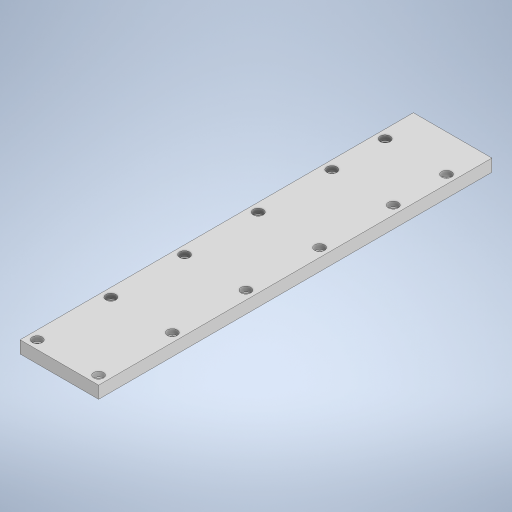
# Autodesk Inventor part: body_cover_v2
Saved by Autodesk Inventor 2023 (Build 270158000, 158)
## iProperties
Created: 2023-07-18
Part Number: body_cover_v2
Material: Generic
Document SubType Name: Modeling
Designer: checo
Density: 1 g/cm^3
Appearance: Default
Author: checo
Autodesk Inventor part; units mm, degrees
ref_plane "YZ Plane" through (0, 0, 0) normal (1, 0, 0) x (0, 1, 0)
ref_plane "XZ Plane" through (0, 0, 0) normal (0, 1, 0) x (-1, 0, 0)
ref_plane "XY Plane" through (0, 0, 0) normal (0, 0, 1) x (1, 0, 0)
sketch "Sketch1" plane through (0, 0, 0) normal (0, 1, 0) x (-1, 0, 0)
  line L0 (-16, -80.1) -> (16, -80.1)
  line L1 (16, -80.1) -> (16, 80.1)
  line L2 (16, 80.1) -> (-16, 80.1)
  line L3 (-16, 80.1) -> (-16, -80.1)
  line L4 (-16, -80.1) -> (16, 80.1) construction
  line L5 (16, -80.1) -> (-16, 80.1) construction
  point P0 (0, 0)
  dimension "d0" = 160.2
  dimension "d1" = 32
  constraints: 12 end point, 2 midpoint, 2 parallel, 1 horizontal, 1 perpendicular
  measures "d0" distance of L0.end L1.end
  measures "d1" distance of L1.end L2.end
extrude "Extrusion1" add sketch "Sketch1" along normal blind 5
sketch "Sketch2" plane through (0, 5, 0) normal (0, 1, 0) x (1, 0, 0)
  line L0 (-16, 80.1) -> (-16, -80.1) projected
  line L1 (-16, -80.1) -> (16, -80.1) projected
  line L2 (0, -80.1) -> (0, 80.1) construction
  line L3 (16, 80.1) -> (-16, 80.1) projected
  point P0 (0, 0)
  point P1 (-12.5, -76.6)
  point P2 (-12.5, -46.6)
  point P3 (-12.5, -16.6)
  point P4 (-12.5, 13.4)
  point P5 (-12.5, 43.4)
  point P6 (-12.5, 65.1)
  point P7 (12.5, -76.6)
  point P8 (12.5, -46.6)
  point P9 (12.5, -16.6)
  point P10 (12.5, 13.4)
  point P11 (12.5, 43.4)
  point P12 (12.5, 65.1)
  dimension "d4" = 3.5
  dimension "d5" = 3.5
  dimension "d8" = 30
  dimension "d13" = 15
  constraints: 6 symmetric about line, 2 end point, 2 midpoint, 1 vertical, 1 vertical alignment, 4 other
  measures "d4" distance from line of point (-12.5, -76.6) L0
  measures "d5" distance from line of point (-12.5, -76.6) L1
  measures "d8" distance of point (-12.5, -76.6) point (-12.5, -46.6)
  measures "d13" distance from line of L3 point (-12.5, 65.1)
hole "Hole1" at (-12.5, 5, 76.6) at (-12.5, 5, 46.6) at (-12.5, 5, 16.6) at (-12.5, 5, -13.4) at (-12.5, 5, -43.4) at (-12.5, 5, -65.1) at (12.5, 5, 76.6) at (12.5, 5, 46.6) at (12.5, 5, 16.6) at (12.5, 5, -13.4) at (12.5, 5, -43.4) at (12.5, 5, -65.1) direction (0, -1, 0) diameter 2.3813 depth 10 tip angle 118 counterbore diameter 4 counterbore depth 2
sketch "Sketch3" plane through (16, 0, -80.1) normal (0, 0, -1) x (-1, 0, 0)
  line L0 (0, 0) -> (0, 5) projected
  line L1 (0, 2.5) -> (32, 2.5) construction
  line L2 (32, 0) -> (32, 5) projected
  line L3 (32, 5) -> (0, 5) construction
  line L4 (16, 5) -> (16, 0) construction
  line L5 (32, 0) -> (0, 0) construction
  point P0 (3, 2.5)
  point P1 (29, 2.5)
  dimension "d22" = 3
  constraints: 4 end point, 3 midpoint, 1 perpendicular, 1 point on line, 1 symmetric about line
  measures "d22" distance from line of L0 point (3, 2.5)
hole "Hole2" at (13, 2.5, -80.1) at (-13, 2.5, -80.1) direction (0, 0, 1) diameter 2.3813 depth 10 tip angle 118
sketch "Sketch6" plane through (0, 0, 0) normal (0, -1, 0) x (1, 0, 0)
  circle A0 centre (12.5, 76.6) radius 1.1906 projected
  line L0 (12.5, 76.6) -> (12.5, -80.6008)
  circle A1 centre (-12.5, 76.6) radius 1.1906 projected
  line L1 (12.5, 76.6) -> (-12.5, 76.6)
  line L2 (-12.5, 76.6) -> (-12.5, -80.1)
  line L3 (16, -80.1) -> (-16, -80.1) projected
  line L4 (11, -80.6008) -> (11, 75.1)
  line L5 (11, 75.1) -> (-11, 75.1)
  line L6 (-11, 75.1) -> (-11, -80.6)
  point P0 (0, 0)
  point P1 (-16, -80.1)
  point P2 (-12.5, 75.4094)
  point P3 (-11.3094, 76.6)
  point P4 (11.3094, 76.6)
  point P5 (12.5, 75.4094)
  point P6 (12.5, -80.1)
  point P7 (11, -80.1)
  point P8 (-11, -80.1)
  dimension "d38" = 1.5
  constraints: 12 end point, 2 perpendicular, 1 vertical, 4 other
  measures "d38" distance between parallel lines of L4 L0
extrude "Extrusion2" cut sketch "Sketch6" against normal blind 0.5 contours A0 L0 L3 L4 L5 L6 L2 A1 L1
fillet "Fillet2" radius 0.5 15 edges at (-12.5, 0.5, -73.1953) (-12.5, 0.5, -54.25) (-12.5, 0.5, -28.4) (-12.5, 0.5, 1.6) (-12.5, 0.5, 31.6) (-12.5, 0.5, 61.6) (0, 0.5, 76.6) (11, 0.5, -2.5) (12.5, 0.5, -73.1953) (12.5, 0.5, -54.25) (12.5, 0.5, -28.4) (12.5, 0.5, 1.6) (12.5, 0.5, 31.6) (12.5, 0.5, 61.6) (-11, 0.5, -2.5)
body "Solid1"
